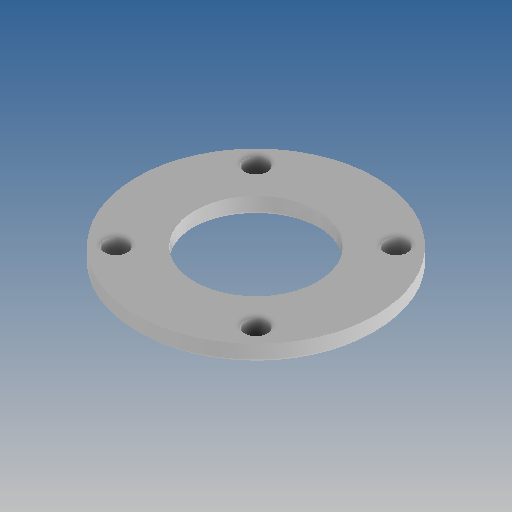
# Autodesk Inventor part: PWTR-0051
Saved by Autodesk Inventor 2021.1 (Build 251245000, 245)
## iProperties
Created: 2020-08-27
Part Number: PWTR-0051
Material: Generic
Document SubType Name: Modeling
Designer: alid
Density: 1 g/cm^3
Appearance: Default
Description: Transfer Case Cover
Author: alid
Revision Number: A
Autodesk Inventor part; units mm, degrees
ref_plane "YZ Plane" through (0, 0, 0) normal (1, 0, 0) x (0, 1, 0)
ref_plane "XZ Plane" through (0, 0, 0) normal (0, 1, 0) x (-1, 0, 0)
ref_plane "XY Plane" through (0, 0, 0) normal (0, 0, 1) x (1, 0, 0)
sketch "Sketch1" plane through (0, 0, 0) normal (0, 0, 1) x (1, 0, 0)
  circle A0 centre (0, 0) radius 35
  circle A1 centre (0, 0) radius 18
  circle A2 centre (0, 0) radius 29 construction
  line L0 (0, 0) -> (0, 29) construction
  line L1 (0, 0) -> (20.5061, 20.5061) construction
  dimension "d0" = 70
  dimension "d1" = 36
  dimension "d2" = 58
  dimension "d3" = 45
  constraints: 4 end point, 3 centre point, 3 coincident, 2 point on circle, 1 vertical
  measures "d0" diameter of A0
  measures "d1" diameter of A1
  measures "d2" diameter of A2
  measures "d3" angle of L1 L0
extrude "Extrusion1" add sketch "Sketch1" along normal blind 5
hole "Hole1" at (20.5061, 20.5061, 0) direction (0, 0, 1) diameter 6.6 end through all clearance for "Countersunk Flat Head Screw ISO 2009/7046" size "M6" standard "ISO"
pattern_circular "Circular Pattern1" count 4 over 360 about axis through (0, 0, -10) along (0, 0, 1) of "Hole1"
chamfer "Chamfer1" distance 1 angle 45 2 edges at (-18, 0, 0) (-35, 0, 0)
body "Solid1"
